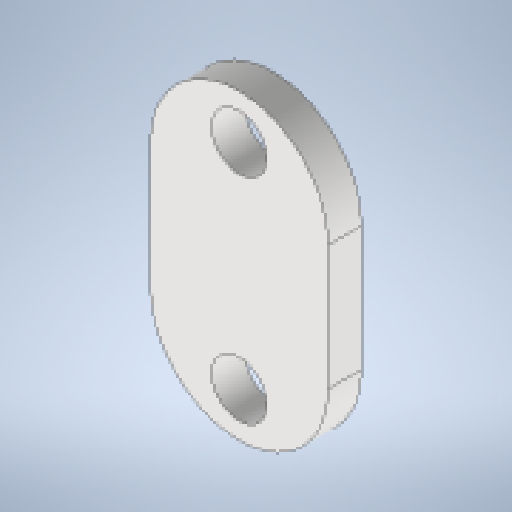
# Autodesk Inventor part: link2part4
Saved by Autodesk Inventor 2024 (Build 280153000, 153)
## iProperties
Created: 2025-02-07
Part Number: link2part4
Material: 一般
Document SubType Name: Modeling
Designer: tanoue_kota
Mass: 0.308093 g
Surface Area: 4.60524 cm^2
Volume: 0.308093 cm^3
Density: 1 g/cm^3
Appearance: 既定
Author: tanoue_kota
Autodesk Inventor part; units mm, degrees
ref_plane "YZ Plane" through (0, 0, 0) normal (1, 0, 0) x (0, 1, 0)
ref_plane "XZ Plane" through (0, 0, 0) normal (0, 1, 0) x (-1, 0, 0)
ref_plane "XY Plane" through (0, 0, 0) normal (0, 0, 1) x (1, 0, 0)
sketch "スケッチ1" plane through (0, 0, 0) normal (0, 0, 1) x (1, 0, 0)
  line L0 (0, 0) -> (10, 0)
  line L1 (10, 0) -> (10, 17)
  line L2 (10, 17) -> (0, 17)
  line L3 (0, 17) -> (0, 0)
  dimension "d0" = 17
  dimension "d1" = 10
  constraints: 8 end point, 2 parallel, 1 horizontal, 1 perpendicular
  measures "d0" distance of L0.end L1.end
  measures "d1" distance of L1.end L2.end
extrude "押し出し1" add sketch "スケッチ1" along normal blind 1.885
sketch "スケッチ2" plane through (0, 0, 1.885) normal (0, 0, 1) x (1, 0, 0)
  line L0 (0, 17) -> (0, 0) projected
  line L1 (0, 8.5) -> (10, 8.5)
  line L2 (10, 0) -> (10, 17) projected
  line L3 (10, 17) -> (0, 17) projected
  line L4 (5, 17) -> (5, 0)
  line L5 (0, 0) -> (10, 0) projected
  line L6 (0, 17) -> (10, 17)
  point P0 (5, 14.5)
  point P1 (5, 2.5)
  dimension "d4" = 6
  constraints: 6 end point, 4 midpoint, 1 point on line, 1 symmetric about line
  measures "d4" distance from line of L1 point (5, 14.5)
hole "穴1" at (5, 14.5, 1.885) at (5, 2.5, 1.885) direction (0, 0, -1) diameter 3.1 end through all
fillet "フィレット1" radius 5 4 edges at (0, 17, 0.9425) (10, 17, 0.9425) (10, 0, 0.9425) (0, 0, 0.9425)
